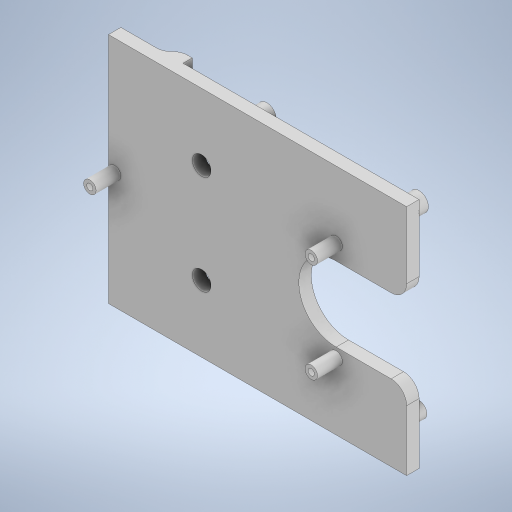
# Autodesk Inventor part: RP4_LidarHolder
Saved by Autodesk Inventor 2024 (Build 280153000, 153)
## iProperties
Created: 2025-05-18
Part Number: RP4_LidarHolder
Material: Ogólny
Document SubType Name: Modeling
Designer: Victoria
Density: 1 g/cm^3
Appearance: Domyślna
Author: Victoria
Autodesk Inventor part; units mm, degrees
ref_plane "YZ Plane" through (0, 0, 0) normal (1, 0, 0) x (0, 1, 0)
ref_plane "XZ Plane" through (0, 0, 0) normal (0, 1, 0) x (-1, 0, 0)
ref_plane "XY Plane" through (0, 0, 0) normal (0, 0, 1) x (1, 0, 0)
sketch "Szkic1" plane through (0, 0, 0) normal (0, 0, 1) x (1, 0, 0)
  line L0 (0, 0) -> (80, 0)
  line L1 (80, 0) -> (80, 75)
  line L2 (80, 75) -> (0, 75)
  line L3 (0, 75) -> (0, 0)
  circle A0 centre (14, 53.5) radius 3
  line L4 (14, 53.5) -> (14, 21.5)
  circle A1 centre (14, 21.5) radius 3
  line L5 (0, 75) -> (-16, 75)
  line L6 (-16, 75) -> (-16, 0)
  line L7 (-16, 0) -> (0, 0)
  line L8 (0, 0) -> (0, 75)
  dimension "d0" = 80
  dimension "d1" = 75
  dimension "d2" = 6
  dimension "d3" = 32
  dimension "d4" = 6
  dimension "d5" = 16
  dimension "d43" = 66
  constraints: 18 end point, 4 parallel, 2 centre point, 2 horizontal, 2 perpendicular, 1 coincident, 1 vertical
  measures "d0" distance of L2.end L1.end
  measures "d1" distance of L1.end L0.end
  measures "d2" diameter of A0
  measures "d3" distance of L4.start L4.end
  measures "d4" diameter of A1
  measures "d5" distance of L7.end L6.end
  measures "d43" distance between parallel lines of L1 L4
extrude "Wyciągnięcie proste1" add sketch "Szkic1" along normal blind 4
sketch "Szkic2" plane through (0, 0, 0) normal (0, 0, -1) x (-1, 0, 0)
  line L0 (16, 75) -> (16, 0) projected
  line L1 (-80, 75) -> (16, 75) projected
  line L2 (-80, 0) -> (-80, 75) projected
  line L3 (16, 0) -> (-80, 0) projected
  circle A0 centre (-14, 53.5) radius 3 projected
  circle A1 centre (-14, 21.5) radius 3 projected
  line L4 (-80, 75) -> (16, 75) projected
  line L5 (0, 0) -> (-4, 0)
  line L6 (-4, 0) -> (-4, 75)
  line L7 (-4, 75) -> (0, 75)
  line L8 (0, 75) -> (0, 0)
  line L9 (-4, 0) -> (-24, 0)
  line L10 (-24, 0) -> (-24, 75)
  line L11 (-24, 75) -> (-4, 75)
  line L12 (-4, 75) -> (-4, 0)
  line L13 (-24.5, 75) -> (-80.5, 75)
  line L14 (-80.5, 75) -> (-80.5, 13.5)
  line L15 (-80.5, 13.5) -> (-24.5, 13.5)
  line L16 (-24.5, 13.5) -> (-24.5, 75)
  line L17 (-28, 17) -> (-77, 17)
  line L18 (-77, 17) -> (-77, 71.5)
  line L19 (-77, 71.5) -> (-28, 71.5)
  line L20 (-28, 71.5) -> (-28, 17)
  circle A2 centre (-28, 71.5) radius 1
  circle A3 centre (-77, 71.5) radius 1
  circle A4 centre (-28, 71.5) radius 3
  circle A5 centre (-77, 71.5) radius 3
  circle A6 centre (-28, 13.5) radius 1
  circle A7 centre (-77, 13.5) radius 1
  circle A8 centre (-77, 13.5) radius 2.5
  circle A9 centre (-28, 13.5) radius 2.5
  dimension "d8" = 4
  dimension "d9" = 20
  dimension "d10" = 56
  dimension "d11" = 61.5
  dimension "d12" = 3.5
  dimension "d15" = 2
  dimension "d16" = 2
  dimension "d19" = 2
  dimension "d20" = 2
  dimension "d34" = 2
  dimension "d35" = 2
  dimension "d36" = 1.5
  dimension "d37" = 1.5
  dimension "d44" = 4
  constraints: 32 end point, 8 centre point, 8 parallel, 5 point on line, 4 perpendicular, 3 horizontal, 2 coincident, 3 other
  measures "d8" distance of L6.end L7.end
  measures "d9" distance of L10.end L11.end
  measures "d10" distance of L15.end L14.end
  measures "d11" distance of L14.end L13.end
  measures "d12" distance between parallel lines of L15 L17
  measures "d15" diameter of A2
  measures "d16" diameter of A3
  measures "d19" radial gap between concentric circles of A2 A4
  measures "d20" radial gap between concentric circles of A3 A5
  measures "d34" diameter of A6
  measures "d35" diameter of A7
  measures "d36" radial gap between concentric circles of A7 A8
  measures "d37" radial gap between concentric circles of A6 A9
  measures "d44" distance from line of L10 L19.end
extrude "Wyciągnięcie proste2" add sketch "Szkic2" along normal blind 3 contours L8 L3 L6 L1 | A5 L19 A3 L18 | A9 L15 A6 | L15 A6 A9 | A8 L15 A7 | L15 A7 A8 | A5 L18 A3 L19 | A4 L20 A2 L19 | L19 A2 L20 A4
sketch "Szkic3" plane through (0, 0, 4) normal (0, 0, 1) x (1, 0, 0)
  circle A0 centre (-14, 37.5) radius 2
  circle A1 centre (-14, 37.5) radius 1
  line L0 (-14, 37.5) -> (57.3, 37.5)
  line L1 (57.3, 37.5) -> (57.3, 53.5)
  line L2 (57.3, 37.5) -> (57.3, 21.5)
  circle A2 centre (57.3, 21.5) radius 1
  circle A3 centre (57.3, 21.5) radius 2
  circle A4 centre (57.3, 53.5) radius 1
  circle A5 centre (57.3, 53.5) radius 2
  point P0 (0, 0)
  dimension "d23" = 4
  dimension "d24" = 2
  dimension "d25" = 71.3
  dimension "d26" = 16
  dimension "d27" = 16
  dimension "d28" = 2
  dimension "d29" = 4
  dimension "d30" = 2
  dimension "d31" = 4
  constraints: 6 centre point, 6 end point, 5 coincident, 1 horizontal, 1 perpendicular, 1 vertical
  measures "d23" diameter of A0
  measures "d24" diameter of A1
  measures "d25" distance of L0.start L0.end
  measures "d26" distance of L0.end L1.end
  measures "d27" distance of L0.end L2.end
  measures "d28" diameter of A2
  measures "d29" diameter of A3
  measures "d30" diameter of A4
  measures "d31" diameter of A5
extrude "Wyciągnięcie proste3" add sketch "Szkic3" along normal blind 8
sketch "Szkic4" plane through (0, 0, 4) normal (0, 0, 1) x (1, 0, 0)
  circle A0 centre (28, 71.5) radius 3 projected
  circle A1 centre (77, 13.5) radius 2.5 projected
  circle A2 centre (28, 13.5) radius 2.5 projected
  line L0 (4, 0) -> (4, 75) projected
  line L1 (80, 75) -> (4, 75) projected
  line L2 (80, 71.5) -> (80, 75) projected
  circle A3 centre (77, 71.5) radius 3 projected
  line L3 (80, 0) -> (80, 71.5) projected
  line L4 (4, 0) -> (80, 0) projected
  circle A4 centre (14, 53.5) radius 3 projected
  circle A5 centre (14, 21.5) radius 3 projected
  circle A6 centre (57.3, 21.5) radius 2 projected
  circle A7 centre (57.3, 53.5) radius 2 projected
  line L5 (57.3, 23.5) -> (57.3, 51.5)
  line L6 (57.3, 51.5) -> (57.3, 36.5)
  line L7 (57.3, 36.5) -> (80, 36.5)
  arc A8 (57.3, 48.5) -> (57.3, 24.5) centre (57.3, 36.5) ccw
  line L8 (57.3, 24.5) -> (80, 24.5)
  line L9 (57.3, 48.5) -> (80, 48.5)
  point P0 (0, 0)
  dimension "d38" = 15
  constraints: 10 end point, 6 point on line, 3 perpendicular, 2 point on circle, 2 vertical alignment, 1 centre point, 1 coincident, 1 horizontal alignment, 2 other
  measures "d38" distance of L5.end L6.end
extrude "Wyciągnięcie proste4" cut sketch "Szkic4" against normal blind 4 contours L8 L5 L7 L3 | L7 L5 L9 L3 | A8 L5
fillet "Zaokrąglenie1" radius 5 2 edges at (80, 24.5, 2) (80, 48.5, 2)
fillet "Zaokrąglenie2" radius 5 2 edges at (0, 37.5, 0) (0, 37.5, -3)
